Autodesk Inventor part; units mm, degrees
(part 3 of 3)
  line L496 (-25.2203, -73.2264) -> (-25.2203, -70.1764)
  line L497 (-25.2203, -70.1764) -> (-23.2705, -70.1764)
  line L498 (-20.8351, -70.8969) -> (-21.2535, -71.0157)
  spline S454 degree 2 poles (-21.2535, -71.0157) (-21.4084, -70.4889) (-21.8552, -70.4889) knots 0 0 0 1 1 1
  spline S455 degree 2 poles (-21.8552, -70.4889) (-22.1341, -70.4889) (-22.2839, -70.6258) knots 0 0 0 1 1 1
  spline S456 degree 2 poles (-22.2839, -70.6258) (-22.4105, -70.742) (-22.4105, -70.9279) knots 0 0 0 1 1 1
  spline S457 degree 2 poles (-22.4105, -70.9279) (-22.4105, -71.1604) (-22.271, -71.274) knots 0 0 0 1 1 1
  spline S458 degree 2 poles (-22.271, -71.274) (-22.1419, -71.3799) (-21.8294, -71.4573) knots 0 0 0 1 1 1
  line L499 (-21.8294, -71.4573) -> (-21.7029, -71.4935)
  spline S459 degree 2 poles (-21.7029, -71.4935) (-21.1399, -71.6381) (-20.9281, -71.9429) knots 0 0 0 1 1 1
  spline S460 degree 2 poles (-20.9281, -71.9429) (-20.7783, -72.0694) (-20.7783, -72.3974) knots 0 0 0 1 1 1
  spline S461 degree 2 poles (-20.7783, -72.3974) (-20.7783, -72.8287) (-21.1579, -73.0792) knots 0 0 0 1 1 1
  spline S462 degree 2 poles (-21.1579, -73.0792) (-21.3749, -73.2832) (-21.8423, -73.2832) knots 0 0 0 1 1 1
  spline S463 degree 2 poles (-21.8423, -73.2832) (-22.2994, -73.2832) (-22.5913, -73.0611) knots 0 0 0 1 1 1
  spline S464 degree 2 poles (-22.5913, -73.0611) (-22.8495, -72.8623) (-22.9554, -72.4723) knots 0 0 0 1 1 1
  line L500 (-22.9554, -72.4723) -> (-22.537, -72.3328)
  spline S465 degree 2 poles (-22.537, -72.3328) (-22.457, -72.6557) (-22.2349, -72.8235) knots 0 0 0 1 1 1
  spline S466 degree 2 poles (-22.2349, -72.8235) (-22.0825, -72.9191) (-21.8501, -72.9191) knots 0 0 0 1 1 1
  spline S467 degree 2 poles (-21.8501, -72.9191) (-21.5092, -72.9191) (-21.3465, -72.7641) knots 0 0 0 1 1 1
  spline S468 degree 2 poles (-21.3465, -72.7641) (-21.2173, -72.6427) (-21.2173, -72.4361) knots 0 0 0 1 1 1
  spline S469 degree 2 poles (-21.2173, -72.4361) (-21.2173, -72.2011) (-21.3516, -72.0901) knots 0 0 0 1 1 1
  spline S470 degree 2 poles (-21.3516, -72.0901) (-21.4885, -71.9713) (-21.863, -71.8731) knots 0 0 0 1 1 1
  line L501 (-21.863, -71.8731) -> (-21.9844, -71.837)
  spline S471 degree 2 poles (-21.9844, -71.837) (-22.4854, -71.7001) (-22.6894, -71.4031) knots 0 0 0 1 1 1
  spline S472 degree 2 poles (-22.6894, -71.4031) (-22.8418, -71.2766) (-22.8418, -70.9434) knots 0 0 0 1 1 1
  spline S473 degree 2 poles (-22.8418, -70.9434) (-22.8418, -70.5741) (-22.5577, -70.3417) knots 0 0 0 1 1 1
  spline S474 degree 2 poles (-22.5577, -70.3417) (-22.2891, -70.1247) (-21.863, -70.1247) knots 0 0 0 1 1 1
  spline S475 degree 2 poles (-21.863, -70.1247) (-21.0727, -70.1247) (-20.8351, -70.8969) knots 0 0 0 1 1 1
  line L502 (-18.2448, -70.1764) -> (-18.2448, -70.5509)
  line L503 (-18.2448, -70.5509) -> (-19.7634, -70.5509)
  line L504 (-19.7634, -70.5509) -> (-19.7634, -71.4212)
  line L505 (-19.7634, -71.4212) -> (-18.6141, -71.4212)
  line L506 (-18.6141, -71.4212) -> (-18.6141, -71.7957)
  line L507 (-18.6141, -71.7957) -> (-19.7634, -71.7957)
  line L508 (-19.7634, -71.7957) -> (-19.7634, -72.8519)
  line L509 (-19.7634, -72.8519) -> (-18.2164, -72.8519)
  line L510 (-18.2164, -72.8519) -> (-18.2164, -73.2264)
  line L511 (-18.2164, -73.2264) -> (-20.1946, -73.2264)
  line L512 (-20.1946, -73.2264) -> (-20.1946, -70.1764)
  line L513 (-20.1946, -70.1764) -> (-18.2448, -70.1764)
  line L514 (-15.6778, -70.1764) -> (-15.6778, -70.556)
  line L515 (-15.6778, -70.556) -> (-16.6101, -70.556)
  line L516 (-16.6101, -70.556) -> (-16.6101, -73.2264)
  line L517 (-16.6101, -73.2264) -> (-17.0465, -73.2264)
  line L518 (-17.0465, -73.2264) -> (-17.0465, -70.556)
  line L519 (-17.0465, -70.556) -> (-17.9685, -70.556)
  line L520 (-17.9685, -70.556) -> (-17.9685, -70.1764)
  line L521 (-17.9685, -70.1764) -> (-15.6778, -70.1764)
  line L522 (-62.9908, -24.0054) -> (-62.9908, -20.9554)
  line L523 (-62.9908, -20.9554) -> (-60.9295, -20.9554)
  line L524 (-60.9295, -20.9554) -> (-60.9295, -21.5362)
  line L525 (-60.9295, -21.5362) -> (-62.2296, -21.5362)
  line L526 (-62.2296, -21.5362) -> (-62.2296, -22.0726)
  line L527 (-62.2296, -22.0726) -> (-61.0308, -22.0726)
  line L528 (-61.0308, -22.0726) -> (-61.0308, -22.6534)
  line L529 (-61.0308, -22.6534) -> (-62.2296, -22.6534)
  line L530 (-62.2296, -22.6534) -> (-62.2296, -23.4245)
  line L531 (-62.2296, -23.4245) -> (-60.9295, -23.4245)
  line L532 (-60.9295, -23.4245) -> (-60.9295, -24.0054)
  line L533 (-60.9295, -24.0054) -> (-62.9908, -24.0054)
  line L534 (-57.8301, -24.0054) -> (-58.7149, -24.0054)
  line L535 (-58.7149, -24.0054) -> (-59.3032, -23.034)
  line L536 (-59.3032, -23.034) -> (-59.9038, -24.0054)
  line L537 (-59.9038, -24.0054) -> (-60.7515, -24.0054)
  line L538 (-60.7515, -24.0054) -> (-59.7604, -22.4705)
  line L539 (-59.7604, -22.4705) -> (-60.712, -20.9554)
  line L540 (-60.712, -20.9554) -> (-59.8271, -20.9554)
  line L541 (-59.8271, -20.9554) -> (-59.276, -21.8773)
  line L542 (-59.276, -21.8773) -> (-58.71, -20.9554)
  line L543 (-58.71, -20.9554) -> (-57.8622, -20.9554)
  line L544 (-57.8622, -20.9554) -> (-58.8187, -22.4384)
  line L545 (-58.8187, -22.4384) -> (-57.8301, -24.0054)
  line L546 (-56.9526, -24.0054) -> (-56.9526, -21.5362)
  line L547 (-56.9526, -21.5362) -> (-57.8548, -21.5362)
  line L548 (-57.8548, -21.5362) -> (-57.8548, -20.9554)
  line L549 (-57.8548, -20.9554) -> (-55.2843, -20.9554)
  line L550 (-55.2843, -20.9554) -> (-55.2843, -21.5362)
  line L551 (-55.2843, -21.5362) -> (-56.1864, -21.5362)
  line L552 (-56.1864, -21.5362) -> (-56.1864, -24.0054)
  line L553 (-56.1864, -24.0054) -> (-56.9526, -24.0054)
  line L554 (-53.7049, -22.9426) -> (-55.0618, -22.9426)
  line L555 (-55.0618, -22.9426) -> (-55.0618, -22.3741)
  line L556 (-55.0618, -22.3741) -> (-53.7049, -22.3741)
  line L557 (-53.7049, -22.3741) -> (-53.7049, -22.9426)
  spline S476 degree 2 poles (-50.8156, -21.9168) (-50.8156, -22.1294) (-50.9515, -22.515) (-51.0775, -22.6435) knots 0 0 0 1 2 2 2
  spline S477 degree 2 poles (-51.0775, -22.6435) (-51.1542, -22.7251) (-51.342, -22.8585) (-51.4532, -22.9055) knots 0 0 0 1 2 2 2
  spline S478 degree 2 poles (-51.4532, -22.9055) (-51.5669, -22.9525) (-51.8314, -23.0068) (-51.9945, -23.0068) knots 0 0 0 1 2 2 2
  line L558 (-51.9945, -23.0068) -> (-52.3949, -23.0068)
  line L559 (-52.3949, -23.0068) -> (-52.3949, -24.0054)
  line L560 (-52.3949, -24.0054) -> (-53.1611, -24.0054)
  line L561 (-53.1611, -24.0054) -> (-53.1611, -20.9554)
  line L562 (-53.1611, -20.9554) -> (-51.9772, -20.9554)
  spline S479 degree 2 poles (-51.9772, -20.9554) (-51.7152, -20.9554) (-51.3321, -21.0518) (-51.1764, -21.1556) knots 0 0 0 1 2 2 2
  spline S480 degree 2 poles (-51.1764, -21.1556) (-51.0034, -21.2718) (-50.8156, -21.6524) (-50.8156, -21.9168) knots 0 0 0 1 2 2 2
  spline S481 degree 2 poles (-51.6015, -21.9366) (-51.6015, -21.8056) (-51.7251, -21.6203) (-51.8091, -21.5856) knots 0 0 0 1 2 2 2
  spline S482 degree 2 poles (-51.8091, -21.5856) (-51.9179, -21.5387) (-52.1156, -21.5239) (-52.2862, -21.5239) knots 0 0 0 1 2 2 2
  line L563 (-52.2862, -21.5239) -> (-52.3949, -21.5239)
  line L564 (-52.3949, -21.5239) -> (-52.3949, -22.4384)
  line L565 (-52.3949, -22.4384) -> (-52.3406, -22.4384)
  spline S483 degree 2 poles (-52.3406, -22.4384) (-52.2343, -22.4384) (-52.0415, -22.4334) (-51.9698, -22.4211) knots 0 0 0 1 2 2 2
  spline S484 degree 2 poles (-51.9698, -22.4211) (-51.908, -22.4112) (-51.7721, -22.3519) (-51.735, -22.3148) knots 0 0 0 1 2 2 2
  spline S485 degree 2 poles (-51.735, -22.3148) (-51.6559, -22.2406) (-51.6015, -22.075) (-51.6015, -21.9366) knots 0 0 0 1 2 2 2
  spline S486 degree 2 poles (-47.6296, -22.4804) (-47.6296, -23.2219) (-48.4205, -24.0696) (-49.1076, -24.0696) knots 0 0 0 1 2 2 2
  spline S487 degree 2 poles (-49.1076, -24.0696) (-49.7972, -24.0696) (-50.5832, -23.212) (-50.5832, -22.4804) knots 0 0 0 1 2 2 2
  spline S488 degree 2 poles (-50.5832, -22.4804) (-50.5832, -21.7463) (-49.7972, -20.8911) (-49.1076, -20.8911) knots 0 0 0 1 2 2 2
  spline S489 degree 2 poles (-49.1076, -20.8911) (-48.4205, -20.8911) (-47.6296, -21.7414) (-47.6296, -22.4804) knots 0 0 0 1 2 2 2
  spline S490 degree 2 poles (-48.4205, -22.4804) (-48.4205, -22.206) (-48.5318, -21.8229) (-48.6282, -21.7018) knots 0 0 0 1 2 2 2
  spline S491 degree 2 poles (-48.6282, -21.7018) (-48.7245, -21.5758) (-48.9717, -21.467) (-49.1052, -21.467) knots 0 0 0 1 2 2 2
  spline S492 degree 2 poles (-49.1052, -21.467) (-49.2461, -21.467) (-49.4759, -21.5683) (-49.5822, -21.6969) knots 0 0 0 1 2 2 2
  spline S493 degree 2 poles (-49.5822, -21.6969) (-49.6761, -21.8155) (-49.7923, -22.2085) (-49.7923, -22.4804) knots 0 0 0 1 2 2 2
  spline S494 degree 2 poles (-49.7923, -22.4804) (-49.7923, -22.7621) (-49.6811, -23.1329) (-49.5847, -23.2589) knots 0 0 0 1 2 2 2
  spline S495 degree 2 poles (-49.5847, -23.2589) (-49.4883, -23.385) (-49.2386, -23.4938) (-49.1052, -23.4938) knots 0 0 0 1 2 2 2
  spline S496 degree 2 poles (-49.1052, -23.4938) (-48.9692, -23.4938) (-48.7171, -23.3776) (-48.6257, -23.254) knots 0 0 0 1 2 2 2
  spline S497 degree 2 poles (-48.6257, -23.254) (-48.5268, -23.1205) (-48.4205, -22.7671) (-48.4205, -22.4804) knots 0 0 0 1 2 2 2
  line L566 (-43.2425, -20.9554) -> (-44.0136, -24.0054)
  line L567 (-44.0136, -24.0054) -> (-44.854, -24.0054)
  line L568 (-44.854, -24.0054) -> (-45.3433, -22.1195)
  line L569 (-45.3433, -22.1195) -> (-45.8154, -24.0054)
  line L570 (-45.8154, -24.0054) -> (-46.6583, -24.0054)
  line L571 (-46.6583, -24.0054) -> (-47.4294, -20.9554)
  line L572 (-47.4294, -20.9554) -> (-46.6335, -20.9554)
  line L573 (-46.6335, -20.9554) -> (-46.2134, -22.997)
  line L574 (-46.2134, -22.997) -> (-45.7042, -20.9554)
  line L575 (-45.7042, -20.9554) -> (-44.9429, -20.9554)
  line L576 (-44.9429, -20.9554) -> (-44.4585, -22.9994)
  line L577 (-44.4585, -22.9994) -> (-44.0185, -20.9554)
  line L578 (-44.0185, -20.9554) -> (-43.2425, -20.9554)
  line L579 (-42.8643, -24.0054) -> (-42.8643, -20.9554)
  line L580 (-42.8643, -20.9554) -> (-40.8029, -20.9554)
  line L581 (-40.8029, -20.9554) -> (-40.8029, -21.5362)
  line L582 (-40.8029, -21.5362) -> (-42.103, -21.5362)
  line L583 (-42.103, -21.5362) -> (-42.103, -22.0726)
  line L584 (-42.103, -22.0726) -> (-40.9043, -22.0726)
  line L585 (-40.9043, -22.0726) -> (-40.9043, -22.6534)
  line L586 (-40.9043, -22.6534) -> (-42.103, -22.6534)
  line L587 (-42.103, -22.6534) -> (-42.103, -23.4245)
  line L588 (-42.103, -23.4245) -> (-40.8029, -23.4245)
  line L589 (-40.8029, -23.4245) -> (-40.8029, -24.0054)
  line L590 (-40.8029, -24.0054) -> (-42.8643, -24.0054)
  line L591 (-37.4662, -24.0054) -> (-38.398, -24.0054)
  line L592 (-38.398, -24.0054) -> (-39.2458, -22.8857)
  line L593 (-39.2458, -22.8857) -> (-39.5226, -22.8857)
  line L594 (-39.5226, -22.8857) -> (-39.5226, -24.0054)
  line L595 (-39.5226, -24.0054) -> (-40.2839, -24.0054)
  line L596 (-40.2839, -24.0054) -> (-40.2839, -20.9554)
  line L597 (-40.2839, -20.9554) -> (-39.058, -20.9554)
  spline S498 degree 2 poles (-39.058, -20.9554) (-38.8034, -20.9554) (-38.4277, -21.0196) (-38.267, -21.1185) knots 0 0 0 1 2 2 2
  spline S499 degree 2 poles (-38.267, -21.1185) (-38.1039, -21.2223) (-37.9111, -21.5461) (-37.9111, -21.7933) knots 0 0 0 1 2 2 2
  spline S500 degree 2 poles (-37.9111, -21.7933) (-37.9111, -22.1418) (-38.2275, -22.5792) (-38.492, -22.7078) knots 0 0 0 1 2 2 2
  line L598 (-38.492, -22.7078) -> (-37.4662, -24.0054)
  spline S501 degree 2 poles (-38.6971, -21.8897) (-38.6971, -21.7735) (-38.7861, -21.6079) (-38.8874, -21.5634) knots 0 0 0 1 2 2 2
  spline S502 degree 2 poles (-38.8874, -21.5634) (-38.9591, -21.5337) (-39.1346, -21.5164) (-39.2656, -21.5164) knots 0 0 0 1 2 2 2
  line L599 (-39.2656, -21.5164) -> (-39.5226, -21.5164)
  line L600 (-39.5226, -21.5164) -> (-39.5226, -22.337)
  line L601 (-39.5226, -22.337) -> (-39.3027, -22.337)
  spline S503 degree 2 poles (-39.3027, -22.337) (-39.1445, -22.337) (-38.9196, -22.2975) (-38.8429, -22.2357) knots 0 0 0 1 2 2 2
  spline S504 degree 2 poles (-38.8429, -22.2357) (-38.7688, -22.1764) (-38.6971, -22.0182) (-38.6971, -21.8897) knots 0 0 0 1 2 2 2
  line L602 (-26.2426, -83.3657) -> (-26.2426, -83.7461)
  line L603 (-26.2426, -83.7461) -> (-27.5586, -83.7461)
  line L604 (-27.5586, -83.7461) -> (-27.5586, -84.7436)
  line L605 (-27.5586, -84.7436) -> (-26.592, -84.7436)
  line L606 (-26.592, -84.7436) -> (-26.592, -85.1174)
  line L607 (-26.592, -85.1174) -> (-27.5586, -85.1174)
  line L608 (-27.5586, -85.1174) -> (-27.5586, -86.4157)
  line L609 (-27.5586, -86.4157) -> (-28.1535, -86.4157)
  line L610 (-28.1535, -86.4157) -> (-28.1535, -83.3657)
  line L611 (-28.1535, -83.3657) -> (-26.2426, -83.3657)
  line L612 (-25.276, -83.3657) -> (-25.276, -86.0419)
  line L613 (-25.276, -86.0419) -> (-23.9247, -86.0419)
  line L614 (-23.9247, -86.0419) -> (-23.9247, -86.4157)
  line L615 (-23.9247, -86.4157) -> (-25.8621, -86.4157)
  line L616 (-25.8621, -86.4157) -> (-25.8621, -83.3657)
  line L617 (-25.8621, -83.3657) -> (-25.276, -83.3657)
  line L618 (-22.2481, -85.7787) -> (-22.9205, -85.7787)
  line L619 (-22.9205, -85.7787) -> (-23.0112, -86.4157)
  line L620 (-23.0112, -86.4157) -> (-23.6017, -86.4157)
  line L621 (-23.6017, -86.4157) -> (-22.9692, -83.3657)
  line L622 (-22.9692, -83.3657) -> (-22.1995, -83.3657)
  line L623 (-22.1995, -83.3657) -> (-21.5647, -86.4157)
  line L624 (-21.5647, -86.4157) -> (-22.1508, -86.4157)
  line L625 (-22.1508, -86.4157) -> (-22.2481, -85.7787)
  line L626 (-22.8652, -85.3961) -> (-22.3057, -85.3961)
  line L627 (-22.3057, -85.3961) -> (-22.5556, -83.7461)
  line L628 (-22.5556, -83.7461) -> (-22.6153, -83.7461)
  line L629 (-22.6153, -83.7461) -> (-22.8652, -85.3961)
  line L630 (-19.4392, -83.3657) -> (-19.4392, -83.7461)
  line L631 (-19.4392, -83.7461) -> (-20.4323, -83.7461)
  spline S505 degree 2 poles (-20.4323, -83.7461) (-20.4964, -83.7461) (-20.596, -83.8147) (-20.6623, -83.9341) (-20.6977, -84.089) (-20.6977, -84.1774) knots 0 0 0 1 2 3 4 4 4
  spline S506 degree 2 poles (-20.6977, -84.1774) (-20.6977, -84.3743) (-20.5539, -84.6154) (-20.4323, -84.6154) knots 0 0 0 1 2 2 2
  line L632 (-20.4323, -84.6154) -> (-19.9236, -84.6154)
  spline S507 degree 2 poles (-19.9236, -84.6154) (-19.7688, -84.6154) (-19.5343, -84.7436) (-19.3751, -84.9692) (-19.2977, -85.2833) (-19.2977, -85.4691) knots 0 0 0 1 2 3 4 4 4
  spline S508 degree 2 poles (-19.2977, -85.4691) (-19.2977, -85.6681) (-19.3839, -86.011) (-19.541, -86.2675) (-19.7599, -86.4157) (-19.8926, -86.4157) knots 0 0 0 1 2 3 4 4 4
  line L633 (-19.8926, -86.4157) -> (-21.1533, -86.4157)
  line L634 (-21.1533, -86.4157) -> (-21.1533, -86.0419)
  line L635 (-21.1533, -86.0419) -> (-20.1381, -86.0419)
  spline S509 degree 2 poles (-20.1381, -86.0419) (-20.0696, -86.0419) (-19.9656, -85.9623) (-19.8904, -85.8274) (-19.8506, -85.6416) (-19.8506, -85.5354) knots 0 0 0 1 2 3 4 4 4
  spline S510 degree 2 poles (-19.8506, -85.5354) (-19.8506, -85.4116) (-19.8926, -85.2369) (-19.9944, -85.1351) (-20.1603, -85.0909) (-20.2885, -85.0909) knots 0 0 0 1 2 3 4 4 4
  line L636 (-20.2885, -85.0909) -> (-20.6181, -85.0909)
  spline S511 degree 2 poles (-20.6181, -85.0909) (-20.7729, -85.0909) (-21.014, -84.967) (-21.1777, -84.7436) (-21.2595, -84.434) (-21.2595, -84.2438) knots 0 0 0 1 2 3 4 4 4
  spline S512 degree 2 poles (-21.2595, -84.2438) (-21.2595, -84.0646) (-21.1777, -83.7417) (-21.0251, -83.5051) (-20.8105, -83.3657) (-20.6778, -83.3657) knots 0 0 0 1 2 3 4 4 4
  line L637 (-20.6778, -83.3657) -> (-19.4392, -83.3657)
  line L638 (-18.371, -83.3657) -> (-18.371, -84.6972)
  line L639 (-18.371, -84.6972) -> (-17.5526, -84.6972)
  line L640 (-17.5526, -84.6972) -> (-17.5526, -83.3657)
  line L641 (-17.5526, -83.3657) -> (-16.9709, -83.3657)
  line L642 (-16.9709, -83.3657) -> (-16.9709, -86.4157)
  line L643 (-16.9709, -86.4157) -> (-17.5526, -86.4157)
  line L644 (-17.5526, -86.4157) -> (-17.5526, -85.071)
  line L645 (-17.5526, -85.071) -> (-18.371, -85.071)
  line L646 (-18.371, -85.071) -> (-18.371, -86.4157)
  line L647 (-18.371, -86.4157) -> (-18.9681, -86.4157)
  line L648 (-18.9681, -86.4157) -> (-18.9681, -83.3657)
  line L649 (-18.9681, -83.3657) -> (-18.371, -83.3657)
  point P0 (0, 0)
  dimension "d40" = 2
  dimension "d41" = 2
  dimension "d42" = 5
  dimension "d43" = 10
  constraints: 8 other
  measures "d40" distance between parallel lines of L9 L8
  measures "d41" distance between parallel lines of L14 L10
  measures "d42" distance between parallel lines of L19 L18
  measures "d43" distance between parallel lines of L20 L15
extrude "Extrusion12" cut sketch "Sketch11" against normal blind 10 contours S0 S1 L21 L22 L23 S2 S3 L24 L25 L26 | L27 L28 S4 S5 L29 L30 L31 L32 L33 L34 S6 S7 L35 | L36 L37 L38 L39 | S8 S9 S10 S11 | L40 L41 L42 L43 L44 S12 L45 S13 L46 L47 | L48 S14 S15 L49 S16 S17 S18 S19 L50 | S22 S23 L52 L53 L54 L55 L56 L57 S24 S25 L58 | L59 S26 S27 S28 S29 S30 S31 L60 S32 S33 S34 S35 S36 S37 | L61 L62 L63 L64 | S38 S39 S40 S41 | L65 L66 L67 S42 S43 S44 S45 L68 L69 L70 L71 | L73 L74 L75 S50 S51 S52 L76 S53 S54 L77 S55 S56 L78 | L81 L82 L83 S60 S61 S62 S63 L84 L85 L86 L87 | L89 L90 L91 S68 S69 S70 S71 L92 L93 L94 L95 | L97 S76 S77 L98 S78 S79 S80 S81 L99 | L101 L102 L103 L104 | L105 L106 L107 L108 L109 S84 L110 S85 L111 L112 | L113 L114 L115 S86 S87 S88 L116 S89 S90 L117 S91 S92 L118 | L121 L122 L123 L124 | L125 L126 L127 L128 | L129 S96 S97 L130 S98 S99 S100 S101 L131 | L133 L134 L135 S104 S105 S106 S107 L136 L137 L138 L139 | L141 S112 S113 L142 S114 S115 S116 S117 L143 | S120 S121 S122 S123 L145 S124 S125 S126 S127 L146 L147 L148 L149 L150 | L151 L152 L153 S128 S129 L154 L155 L156 S130 S131 L157 L158 L159 | L160 L161 L162 S132 S133 S134 L163 S135 S136 L164 S137 S138 L165 | S142 S143 L168 L169 L170 L171 L172 L173 L174 L175 L176 L177 L178 S144 S145 L179 | L180 S146 S147 L181 S148 S149 S150 S151 L182 | L184 L185 S154 S155 L186 L187 L188 S156 S157 L189 L190 L191 L192 L193 L194 S158 S159 S160 S161 L195 | L196 L197 L198 S162 S163 S164 L199 S165 S166 L200 S167 S168 L201 | L204 L205 L206 L207 | L208 L209 L210 S172 S173 S174 L211 S175 S176 L212 S177 S178 L213 | L216 L217 L218 L219 L220 S182 L221 S183 L222 L223 | L224 L225 L226 S184 S185 S186 L227 S187 S188 L228 S189 S190 L229 | S194 S195 L232 L233 L234 L235 L236 L237 S196 S197 L238 | L239 L240 L241 L242 | S198 S199 S200 S201 | L243 L244 L245 L246 | L247 L248 L249 L250 | L251 L252 L253 S202 S203 S204 L254 S205 S206 L255 S207 S208 L256 | L259 L260 L261 L262 L263 L264 L265 L266 L267 L268 L269 L270 | L271 S212 S213 S214 S215 S216 S217 L272 S218 S219 S220 S221 S222 S223 | S224 S225 L273 L274 L275 L276 L277 L278 L279 L280 L281 L282 L283 S226 S227 L284 | L285 L286 L287 L288 | S228 S229 S230 S231 | L289 L290 S232 S233 L291 L292 L293 S234 S235 L294 L295 L296 L297 L298 L299 S236 S237 S238 S239 L300 | L301 L302 L303 S240 S241 L304 L305 L306 S242 S243 L307 L308 L309 | L310 L311 L312 L313 | L314 L315 L316 S244 S245 S246 L317 S247 S248 L318 S249 S250 L319 | L322 L323 L324 S254 S255 S256 S257 L325 L326 L327 L328 | S262 S263 S264 S265 | S270 S271 L330 L331 L332 L333 L334 L335 S272 S273 L336 | L337 L338 L339 S274 S275 S276 L340 S277 S278 L341 S279 S280 L342 | L345 L346 L347 L348 L349 S284 L350 S285 L351 L352 | L353 L354 S286 L355 S287 L356 L357 L358 L359 L360 S288 L361 S289 L362 L363 L364 | L365 S290 S291 S292 S293 S294 S295 L366 S296 S297 S298 S299 S300 S301 | L367 L368 S302 L369 L370 L371 L372 L373 S303 S304 L374 S305 L375 | S308 S309 S310 S311 | L379 L380 L381 S316 S317 S318 S319 L382 L383 L384 L385 | S324 S325 L387 L388 L389 L390 L391 L392 S326 S327 L393 | L394 L395 L396 L397 | S328 S329 S330 S331 | S332 S333 L398 S334 S335 L399 L400 S336 S337 S338 S339 L401 L402 L403 L404 | S344 S345 S346 S347 | L406 L407 L408 L409 L410 L411 L412 L413 L414 L415 | L416 L417 L418 L419 | S352 S353 S354 S355 | S356 S357 L420 S358 S359 L421 L422 S360 S361 S362 S363 L423 L424 L425 L426 | L428 L429 L430 S368 S369 L431 L432 L433 S370 S371 L434 L435 L436 | L437 S372 S373 L438 S374 S375 S376 S377 L439 | S380 S381 L441 L442 L443 L444 L445 L446 S382 S383 L447 | S384 S385 S386 S387 | L448 L449 L450 S392 S393 S394 L451 S395 S396 L452 S397 S398 L453 | L456 L457 L458 S402 L459 S403 L460 | S404 S405 S406 S407 L461 S408 S409 L462 S410 S411 | L463 L464 L465 S416 L466 S417 L467 | S418 S419 S420 S421 L468 S422 S423 L469 S424 S425 | S430 L470 S431 L471 L472 L473 L474 | S432 S433 S434 S435 S436 S437 S438 S439
extrude "Extrusion13" cut sketch "Sketch11" against normal blind 10 contours L475 S448 S449 S450 L476 L477 L478 L479 L480 L481 L482 | L486 L487 L488 L489 L490 L491 L492 L493 L494 L495 L496 L497 | L498 S454 S455 S456 S457 S458 L499 S459 S460 S461 S462 S463 S464 L500 S465 S466 S467 S468 S469 S470 L501 S471 S472 S473 S474 S475 | L502 L503 L504 L505 L506 L507 L508 L509 L510 L511 L512 L513 | L514 L515 L516 L517 L518 L519 L520 L521
extrude "Extrusion14" cut sketch "Sketch11" against normal blind 10 contours L522 L523 L524 L525 L526 L527 L528 L529 L530 L531 L532 L533 | L534 L535 L536 L537 L538 L539 L540 L541 L542 L543 L544 L545 | L546 L547 L548 L549 L550 L551 L552 L553 | L554 L555 L556 L557 | S476 S477 S478 L558 L559 L560 L561 L562 S479 S480 | S486 S487 S488 S489 | L566 L567 L568 L569 L570 L571 L572 L573 L574 L575 L576 L577 L578 | L579 L580 L581 L582 L583 L584 L585 L586 L587 L588 L589 L590 | L591 L592 L593 L594 L595 L596 L597 S498 S499 S500 L598
extrude "Extrusion15" cut sketch "Sketch11" against normal blind 10 contours L602 L603 L604 L605 L606 L607 L608 L609 L610 L611 | L612 L613 L614 L615 L616 L617 | L618 L619 L620 L621 L622 L623 L624 L625 | L630 L631 S505 S506 L632 S507 S508 L633 L634 L635 S509 S510 L636 S511 S512 L637 | L638 L639 L640 L641 L642 L643 L644 L645 L646 L647 L648 L649
body "Solid1"
